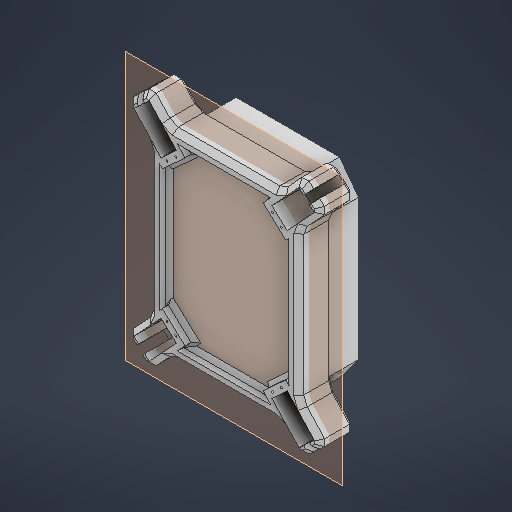
# Autodesk Inventor part: Body
Saved by Autodesk Inventor 2026 (Build 300175050, 175E)
## iProperties
Created: 2026-08-07
Part Number: Body
Material: Generic
Document SubType Name: Modeling
Designer: sidsi
Density: 1 g/cm^3
Appearance: Default
Author: sidsi
Autodesk Inventor part; units mm, degrees
ref_plane "YZ Plane" through (0, 0, 0) normal (1, 0, 0) x (0, 1, 0)
ref_plane "XZ Plane" through (0, 0, 0) normal (0, 1, 0) x (-1, 0, 0)
ref_plane "XY Plane" through (0, 0, 0) normal (0, 0, 1) x (1, 0, 0)
sketch "Sketch1" plane through (0, 0, 0) normal (0, 1, 0) x (-1, 0, 0)
  point P0 (0, 0)
sketch "Sketch2" plane through (0, 0, 0) normal (0, 0, 1) x (1, 0, 0)
  line L0 (0, 0) -> (150, 0)
  line L1 (150, 0) -> (150, 200)
  line L2 (150, 200) -> (0, 200)
  line L3 (0, 200) -> (0, 0)
  line L4 (150.121945, 213.262921) -> (165.542717, 199.008105)
  line L5 (165.542717, 199.008105) -> (138.390688, 169.635205)
  line L6 (138.390688, 169.635205) -> (122.969915, 183.890021)
  line L7 (122.969915, 183.890021) -> (150.121945, 213.262921)
  line L8 (151.541338, 222.164344) -> (174.305335, 201.121521)
  line L9 (174.305335, 201.121521) -> (136.971294, 160.733782)
  line L10 (136.971294, 160.733782) -> (114.207297, 181.776606)
  line L11 (114.207297, 181.776606) -> (151.541338, 222.164344)
  circle A0 centre (132.382247, 169.764649) radius 1
  circle A1 centre (123.559163, 177.898127) radius 1
  line L12 (154.895041, 208.850716) -> (159.986047, 214.358135)
  line L13 (160.769621, 203.42031) -> (165.860627, 208.927729)
  line L14 (0, 100) -> (150, 100)
  line L15 (75, 200) -> (75, 0)
  line L16 (10, 200) -> (10, 0)
  line L17 (0, 10) -> (150, 10)
  line L18 (0, 190) -> (150, 190)
  line L19 (140, 200) -> (140, 0)
  line L20 (-0.121945, 213.262921) -> (-15.542717, 199.008105)
  line L21 (-15.542717, 199.008105) -> (11.609312, 169.635205)
  line L22 (11.609312, 169.635205) -> (27.030085, 183.890021)
  line L23 (27.030085, 183.890021) -> (-0.121945, 213.262921)
  line L24 (-1.541338, 222.164344) -> (-24.305335, 201.121521)
  line L25 (-24.305335, 201.121521) -> (13.028706, 160.733782)
  line L26 (13.028706, 160.733782) -> (35.792703, 181.776606)
  line L27 (35.792703, 181.776606) -> (-1.541338, 222.164344)
  circle A2 centre (17.617753, 169.764649) radius 1
  circle A3 centre (26.440837, 177.898127) radius 1
  line L28 (-4.895041, 208.850716) -> (-9.986047, 214.358135)
  line L29 (-10.769621, 203.42031) -> (-15.860627, 208.927729)
  line L30 (150.121945, -13.262921) -> (165.542717, 0.991895)
  line L31 (165.542717, 0.991895) -> (138.390688, 30.364795)
  line L32 (138.390688, 30.364795) -> (122.969915, 16.109979)
  line L33 (122.969915, 16.109979) -> (150.121945, -13.262921)
  line L34 (151.541338, -22.164344) -> (174.305335, -1.121521)
  line L35 (174.305335, -1.121521) -> (136.971294, 39.266218)
  line L36 (136.971294, 39.266218) -> (114.207297, 18.223394)
  line L37 (114.207297, 18.223394) -> (151.541338, -22.164344)
  circle A4 centre (132.382247, 30.235351) radius 1
  circle A5 centre (123.559163, 22.101873) radius 1
  line L38 (154.895041, -8.850716) -> (159.986047, -14.358135)
  line L39 (160.769621, -3.42031) -> (165.860627, -8.927729)
  line L40 (35.792703, 18.223394) -> (-1.541338, -22.164344)
  line L41 (27.030085, 16.109979) -> (-0.121945, -13.262921)
  line L42 (-4.895041, -8.850716) -> (-9.986047, -14.358135)
  line L43 (-10.769621, -3.42031) -> (-15.860627, -8.927729)
  line L44 (-0.121945, -13.262921) -> (-15.542717, 0.991895)
  line L45 (-1.541338, -22.164344) -> (-24.305335, -1.121521)
  line L46 (-24.305335, -1.121521) -> (13.028706, 39.266218)
  line L47 (-15.542717, 0.991895) -> (11.609312, 30.364795)
  line L48 (13.028706, 39.266218) -> (35.792703, 18.223394)
  circle A6 centre (26.440837, 22.101873) radius 1
  circle A7 centre (17.617753, 30.235351) radius 1
  line L49 (11.609312, 30.364795) -> (27.030085, 16.109979)
  point P0 (150, 174.828157)
  point P1 (131.052829, 200)
  point P2 (18.947171, 200)
  point P3 (0, 174.828157)
  point P4 (0, 25.171843)
  point P5 (18.947171, 0)
  point P6 (131.052829, 0)
  point P7 (150, 25.171843)
  point P8 (140, 35.989782)
  point P9 (121.808924, 10)
  point P10 (28.191076, 10)
  point P11 (10, 35.989782)
  point P12 (10, 164.010218)
  point P13 (28.191076, 190)
  point P14 (121.808924, 190)
  point P15 (140, 164.010218)
  dimension "d0" = 150
  dimension "d1" = 200
  dimension "d2" = 21
  dimension "d3" = 55
  dimension "d4" = 40
  dimension "d5" = 7.5
  dimension "d6" = 5
  dimension "d7" = 5
  dimension "d8" = 2
  dimension "d9" = 2
  dimension "d11" = 4.5
  dimension "d12" = 4
  dimension "d13" = 42.75
  dimension "d14" = 4.5
  dimension "d15" = 6.5
  dimension "d16" = 6.5
  dimension "d17" = 10
  dimension "d18" = 10
  constraints: 100 end point, 46 symmetric about line, 20 point on line, 8 centre point, 7 perpendicular, 6 parallel, 4 midpoint, 1 horizontal, 6 other
  measures "d0" distance of L1.end L2.end
  measures "d1" distance of L0.end L1.end
  measures "d2" distance of L4.start L4.end
  measures "d3" distance of L8.end L9.end
  measures "d4" distance of L4.end L5.end
  measures "d5" distance between parallel lines of L8 L4
  measures "d6" distance between parallel lines of L9 L5
  measures "d7" distance between parallel lines of L7 L11
  measures "d8" diameter of A1
  measures "d9" diameter of A0
  measures "d11" distance from line of L5 A0.centre
  measures "d12" distance from line of L6 A1.centre
  measures "d13" angle of L9 L1
  measures "d14" distance from line of A1.centre L7
  measures "d15" distance between parallel lines of L5 L13
  measures "d16" distance between parallel lines of L7 L12
  measures "d17" distance between parallel lines of L16 L3
  measures "d18" distance between parallel lines of L0 L17
extrude "Extrusion1" add sketch "Sketch2" along normal blind 30 contours L41 L17 L40 L0 | L0 L40 L45 L42 L44 L41 | L47 L44 L43 L45 L46 L3 | L3 L46 L16 L47 | L40 L17 L15 L0 | L41 L49 L47 L16 L46 L48 L40 L17 | L3 L14 L16 L46 | L15 L17 L37 L0 | L3 L25 L16 L14 | L37 L17 L33 L0 | L0 L33 L30 L38 L34 L37 | L25 L24 L29 L20 L21 L3 | L3 L21 L16 L25 | L37 L36 L35 L19 L31 L32 L33 L17 | L16 L21 L22 L23 L18 L27 L26 L25 | L19 L9 L1 L14 | L14 L1 L35 L19 | L18 L27 L2 L15 | L15 L2 L11 L18 | L39 L30 L31 L1 L35 L34 | L19 L5 L1 L9 | L9 L10 L11 L18 L7 L6 L5 L19 | L35 L1 L31 L19 | L18 L23 L2 L27 | L11 L2 L7 L18 | L24 L27 L2 L23 L20 L28 | L1 L5 L4 L13 L8 L9 | L11 L8 L12 L4 L7 L2
sketch "Sketch3" plane through (0, 0, 0) normal (0, 0, -1) x (-1, 0, 0)
  line L0 (0, 174.828157) -> (0, 25.171843)
  line L1 (0, 25.171843) -> (0, 174.828157)
  line L2 (15.860627, 208.927729) -> (24.305335, 201.121521)
  line L3 (0, 174.828157) -> (24.305335, 201.121521)
  line L4 (-18.947171, 200) -> (1.541338, 222.164344)
  line L5 (24.305335, 201.121521) -> (1.541338, 222.164344)
  line L6 (1.541338, 222.164344) -> (-18.947171, 200)
  line L7 (-151.541338, 222.164344) -> (-131.052829, 200)
  line L8 (-18.947171, 200) -> (-131.052829, 200)
  line L9 (-159.986047, 214.358135) -> (-151.541338, 222.164344)
  line L10 (-131.052829, 200) -> (-151.541338, 222.164344)
  line L11 (-151.541338, 222.164344) -> (-174.305335, 201.121521)
  line L12 (-150, 25.171843) -> (-150, 174.828157)
  line L13 (-174.305335, 201.121521) -> (-150, 174.828157)
  line L14 (-174.305335, -1.121521) -> (-150, 25.171843)
  line L15 (-150, 174.828157) -> (-150, 25.171843)
  line L16 (-165.860627, -8.927729) -> (-174.305335, -1.121521)
  line L17 (-150, 25.171843) -> (-174.305335, -1.121521)
  line L18 (-174.305335, -1.121521) -> (-151.541338, -22.164344)
  line L19 (-151.541338, -22.164344) -> (-131.052829, 0)
  line L20 (-131.052829, 0) -> (-18.947171, 0)
  line L21 (-18.947171, 0) -> (1.541338, -22.164344)
  line L22 (1.541338, -22.164344) -> (24.305335, -1.121521)
  line L23 (24.305335, -1.121521) -> (0, 25.171843)
  point P0 (0, 0)
  constraints: 32 end point, 10 perpendicular, 3 parallel, 2 collinear, 1 vertical
extrude "Extrusion2" add sketch "Sketch3" along normal blind 4
sketch "Sketch4" plane through (0, 0, 0) normal (0, 0, 1) x (1, 0, 0)
  line L0 (121.808924, 10) -> (28.191076, 10)
  line L1 (28.191076, 10) -> (35.792703, 18.223394)
  line L2 (13.028706, 39.266218) -> (10, 35.989782)
  line L3 (35.792703, 18.223394) -> (13.028706, 39.266218)
  line L4 (13.028706, 39.266218) -> (10, 35.989782)
  line L5 (10, 35.989782) -> (10, 164.010218)
  line L6 (10, 35.989782) -> (10, 164.010218)
  line L7 (10, 164.010218) -> (13.028706, 161.210511)
  line L8 (10, 164.010218) -> (13.028706, 160.733782)
  line L9 (10, 164.010218) -> (13.028706, 160.733782)
  line L10 (13.028706, 160.733782) -> (35.792703, 181.776606)
  line L11 (35.792703, 181.776606) -> (28.191076, 190)
  line L12 (28.191076, 190) -> (121.808924, 190)
  line L13 (28.191076, 190) -> (121.808924, 190)
  line L14 (121.808924, 190) -> (114.207297, 181.776606)
  line L15 (121.808924, 190) -> (114.207297, 181.776606)
  line L16 (114.207297, 181.776606) -> (136.971294, 160.733782)
  line L17 (136.971294, 160.733782) -> (140, 164.010218)
  line L18 (140, 164.010218) -> (140, 35.989782)
  line L19 (140, 35.989782) -> (136.971294, 39.266218)
  line L20 (136.971294, 39.266218) -> (114.207297, 18.223394)
  line L21 (114.207297, 18.223394) -> (121.808924, 10)
  line L22 (121.808924, 10) -> (28.191076, 10)
  point P0 (0, 0)
  constraints: 34 end point, 9 perpendicular, 5 collinear, 2 parallel
extrude "Extrusion3" cut sketch "Sketch4" against normal blind 4
ref_plane "Work Plane1" through (0, 0, 20) normal (0, 0, 1) x (1, 0, 0)
sketch "Sketch5" plane through (0, 0, 20) normal (0, 0, 1) x (1, 0, 0)
  line L0 (10.647544, 36.690292) -> (13.028706, 39.266218)
  line L1 (13.028706, 39.266218) -> (35.792703, 18.223394)
  line L2 (121.808924, 10) -> (28.191076, 10)
  line L3 (35.792703, 18.223394) -> (28.191076, 10)
  line L4 (28.191076, 10) -> (121.808924, 10)
  line L5 (121.808924, 10) -> (114.207297, 18.223394)
  line L6 (114.207297, 18.223394) -> (136.971294, 39.266218)
  line L7 (136.971294, 39.266218) -> (140, 35.989782)
  line L8 (140, 35.989782) -> (140, 164.010218)
  line L9 (140, 164.010218) -> (136.971294, 160.733782)
  line L10 (136.971294, 160.733782) -> (114.207297, 181.776606)
  line L11 (114.207297, 181.776606) -> (121.808924, 190)
  line L12 (35.792703, 181.776606) -> (28.191076, 190)
  line L13 (121.808924, 190) -> (28.191076, 190)
  line L14 (28.191076, 190) -> (35.792703, 181.776606)
  line L15 (35.792703, 181.776606) -> (13.028706, 160.733782)
  line L16 (13.028706, 160.733782) -> (10, 164.010218)
  line L17 (10, 164.010218) -> (10, 35.989782)
  line L18 (10, 35.989782) -> (10.647211, 36.689931)
  line L19 (114.207297, 181.776606) -> (121.808924, 190)
  line L20 (121.808924, 190) -> (28.191076, 190)
  line L21 (28.191076, 190) -> (35.792703, 181.776606)
  line L22 (35.792703, 181.776606) -> (13.028706, 160.733782)
  line L23 (140, 164.010218) -> (140, 35.989782)
  line L24 (140, 35.989782) -> (136.971294, 39.266218)
  line L25 (136.971294, 39.266218) -> (114.207297, 18.223394)
  line L26 (114.207297, 18.223394) -> (121.808924, 10)
  line L27 (121.808924, 10) -> (28.191076, 10)
  line L28 (28.191076, 10) -> (35.792703, 18.223394)
  line L29 (35.792703, 18.223394) -> (13.028706, 39.266218)
  line L30 (13.028706, 39.266218) -> (10, 35.989782)
  line L31 (10, 164.010218) -> (10, 35.989782)
  line L32 (10, 35.989782) -> (10, 164.010218)
  line L33 (10, 164.010218) -> (13.028706, 160.733782)
  line L34 (13.028706, 160.733782) -> (35.792703, 181.776606)
  line L35 (28.191076, 190) -> (121.808924, 190)
  line L36 (35.792703, 181.776606) -> (28.191076, 190)
  line L37 (28.191076, 190) -> (121.808924, 190)
  line L38 (121.808924, 190) -> (114.207297, 181.776606)
  point P0 (0, 0)
  constraints: 70 end point, 18 perpendicular, 9 collinear, 2 parallel, 1 vertical
extrude "Extrusion4" add sketch "Sketch5" against normal blind 10
chamfer "Chamfer1" distance 5 angle 45 16 edges at (131.0528, 0, 13) (18.9472, 0, 13) (-1.5413, -22.1643, 13) (-24.3053, -1.1215, 13) (0, 25.1718, 13) (0, 174.8282, 13) (-24.3053, 201.1215, 13) (-1.5413, 222.1643, 13) (18.9472, 200, 13) (131.0528, 200, 13) (151.5413, 222.1643, 13) (174.3053, 201.1215, 13) (150, 174.8282, 13) (150, 25.1718, 13) (174.3053, -1.1215, 13) (151.5413, -22.1643, 13)
chamfer "Chamfer2" distance 5 angle 45 36 edges at (75, 200, 30) (19.7502, 201.8358, 30) (8.7029, 211.0822, 30) (130.2498, 201.8358, 30) (141.2971, 211.0822, 30) (157.5995, 216.5642, 30) (168.2472, 206.7216, 30) (162.1527, 187.9748, 30) (151.697, 174.164, 30) (150, 100, 30) (151.697, 25.836, 30) (162.1527, 12.0252, 30) (168.2472, -6.7216, 30) (157.5995, -16.5642, 30) (141.2971, -11.0822, 30) (130.2498, -1.8358, 30) (75, 0, 30) (19.7502, -1.8358, 30) (8.7029, -11.0822, 30) (-7.5995, -16.5642, 30) (-18.2472, -6.7216, 30) (-20.7725, -0.9827, 30) (-12.1527, 12.0252, 30) (151.6801, -18.6315, 30) (170.7725, -0.9827, 30) (170.7725, 200.9827, 30) (151.6801, 218.6315, 30) (-1.6801, 218.6315, 30) (-7.5995, 216.5642, 30) (-18.2472, 206.7216, 30) (-20.7725, 200.9827, 30) (-12.1527, 187.9748, 30) (-1.697, 174.164, 30) (0, 100, 30) (-1.697, 25.836, 30) (-1.6801, -18.6315, 30)
chamfer "Chamfer3" distance 4 angle 45 16 edges at (138.4856, 37.628, 20) (118.0081, 14.1117, 20) (125.5893, 28.7448, 20) (31.9919, 14.1117, 20) (11.5144, 37.628, 20) (11.5144, 162.372, 20) (31.9919, 185.8883, 20) (118.0081, 185.8883, 20) (138.4856, 162.372, 20) (140, 100, 20) (125.5893, 171.2552, 20) (75, 190, 20) (24.4107, 171.2552, 20) (10, 100, 20) (24.4107, 28.7448, 20) (75, 10, 20)
chamfer "Chamfer4" distance 4 angle 45 32 edges at (-12.1527, 12.0252, -4) (-1.697, 25.836, -4) (0, 100, -4) (-1.697, 174.164, -4) (-12.1527, 187.9748, -4) (-20.7725, 200.9827, -4) (-12.9233, 211.6429, -4) (-20.7725, -0.9827, -4) (-12.9233, -11.6429, -4) (-1.6801, -18.6315, -4) (8.7029, -11.0822, -4) (19.7502, -1.8358, -4) (75, 0, -4) (130.2498, -1.8358, -4) (141.2971, -11.0822, -4) (151.6801, -18.6315, -4) (162.9233, -11.6429, -4) (170.7725, -0.9827, -4) (162.1527, 12.0252, -4) (151.697, 25.836, -4) (150, 100, -4) (151.697, 174.164, -4) (162.1527, 187.9748, -4) (170.7725, 200.9827, -4) (162.9233, 211.6429, -4) (151.6801, 218.6315, -4) (141.2971, 211.0822, -4) (130.2498, 201.8358, -4) (75, 200, -4) (19.7502, 201.8358, -4) (8.7029, 211.0822, -4) (-1.6801, 218.6315, -4)
sketch "Sketch6" plane through (0, 0, -4) normal (0, 0, -1) x (-1, 0, 0)
  line L0 (-23.110616, 4) -> (-126.889384, 4)
  line L1 (-126.889384, 4) -> (-23.076426, 4)
  line L2 (-23.076426, 4) -> (-23.076426, 10)
  line L3 (-23.076426, 10) -> (-126.889384, 10)
  line L4 (-126.889384, 10) -> (-126.889384, 4)
  line L5 (-126.889384, 196) -> (-23.110616, 196)
  line L6 (-23.110616, 196) -> (-126.906056, 196)
  line L7 (-126.906056, 196) -> (-126.906056, 190)
  line L8 (-126.906056, 190) -> (-23.110616, 190)
  line L9 (-23.110616, 190) -> (-23.110616, 196)
  line L10 (-28.191076, 10) -> (-121.808924, 10)
  line L11 (-121.808924, 190) -> (-28.191076, 190)
  line L12 (-4, 170.583061) -> (-4, 29.416939)
  line L13 (-4, 29.416939) -> (-10, 29.416939)
  line L14 (-10, 29.416939) -> (-10, 170.630581)
  line L15 (-10, 170.630581) -> (-4, 170.630581)
  line L16 (-4, 170.630581) -> (-4, 29.416939)
  line L17 (-10, 164.010218) -> (-10, 35.989782)
  line L18 (-146, 29.416939) -> (-146, 170.583061)
  line L19 (-146, 29.416939) -> (-140, 29.416939)
  line L20 (-140, 29.416939) -> (-140, 170.611773)
  line L21 (-140, 170.611773) -> (-146, 170.611773)
  line L22 (-146, 170.611773) -> (-146, 29.416939)
  line L23 (-140, 35.989782) -> (-140, 164.010218)
  line L24 (-126.906056, 196) -> (-146, 170.611773)
  line L25 (-146, 170.611773) -> (-140, 166.099301)
  line L26 (-140, 166.099301) -> (-121.808924, 190)
  line L27 (-4, 100.02376) -> (-146, 100.014356)
  line L28 (-74.982905, 4) -> (-75.008336, 196)
  line L29 (-126.893343, 4.031242) -> (-145.990649, 29.41694)
  line L30 (-139.991247, 33.930207) -> (-121.808924, 10)
  line L31 (-10, 34.045425) -> (-10, 35.989782)
  line L32 (-10, 34.045425) -> (-10, 29.416939)
  line L33 (-10, 29.416939) -> (-3.88195, 29.416939)
  line L34 (-4, 170.583061) -> (0, 169.828157)
  line L35 (-23.110616, 196) -> (-13.183731, 200.342109)
  line L36 (-4, 170.583061) -> (-23.110616, 196)
  line L37 (-23.110616, 196) -> (-28.191076, 190)
  line L38 (-28.191076, 190) -> (-10, 165.806041)
  line L39 (-13.183731, -0.342109) -> (-23.110616, 4)
  line L40 (-3.88195, 29.416939) -> (-23.110616, 4)
  line L41 (-23.110616, 4) -> (-28.191076, 10)
  line L42 (-28.191076, 10) -> (-10, 34.045425)
  line L43 (-10, 34.045425) -> (-3.88195, 29.416939)
  line L44 (-139.991247, 33.930207) -> (-145.990649, 29.41694)
  line L45 (-121.808924, 10) -> (-126.893343, 4.031242)
  point P0 (0, 0)
  point P1 (-145.990649, 29.416939)
  point P2 (-126.889384, 4.03589)
  point P3 (-23.076426, 4.045193)
  point P4 (-4.03573, 170.630581)
  point P5 (-140, 33.923622)
  dimension "d41" = 0
  dimension "d42" = 0
  dimension "d43" = 0
  dimension "d44" = 0
  constraints: 70 end point, 10 parallel, 7 perpendicular, 4 horizontal, 4 midpoint, 3 symmetric about line, 2 point on line, 1 collinear
  measures "d41" distance between parallel lines of L10 L3
  measures "d42" distance between parallel lines of L11 L8
  measures "d43" distance between parallel lines of L17 L14
  measures "d44" distance between parallel lines of L23 L20
extrude "Extrusion5" add sketch "Sketch6" along normal blind 30 contours L40 L2 L1 | L41 L3 L2 L40 | L0 L28 L3 L41 | L0 L4 L45 L3 L28 | L2 L3 L42 L14 L13 L33 L40 | L43 L12 L13 L14 | L14 L27 L12 L43 | L45 L29 L19 L20 L44 L30 L3 L4 | L4 L3 L45 | L14 L15 L36 L12 L27 | L27 L18 L22 L25 L20 | L20 L44 L19 L18 L27 | L28 L5 L37 L8 | L8 L7 L6 L5 L28 | L44 L20 L19 | L26 L20 L21 L24 L7 L8 | L37 L9 L8 | L8 L9 L36 L15 L14 L38 | L36 L15 L16 | L25 L21 L20
body "Solid1"
